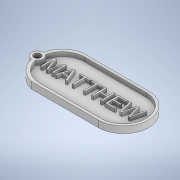
# Autodesk Inventor part: name_tag
Saved by Autodesk Inventor 2020 (Build 240168000, 168)
## iProperties
Created: 2022-11-14
Part Number: name_tag
Material: Generic
Document SubType Name: Modeling
Designer: Matthew Ng
Density: 1 g/cm^3
Appearance: Default
Author: Matthew Ng
Autodesk Inventor part; units mm, degrees
note: some values were not read from the file. Chosen so that the rebuilt part matches the saved one: direction of "Emboss1".
ref_plane "YZ Plane" through (0, 0, 0) normal (1, 0, 0) x (0, 1, 0)
ref_plane "XZ Plane" through (0, 0, 0) normal (0, 1, 0) x (-1, 0, 0)
ref_plane "XY Plane" through (0, 0, 0) normal (0, 0, 1) x (1, 0, 0)
sketch "Sketch1" plane through (0, 0, 0) normal (0, 1, 0) x (-1, 0, 0)
  line L0 (-15, 0) -> (-55, 0)
  line L1 (-55, -30) -> (-15, -30)
  arc A0 (-55, 0) -> (-55, -30) centre (-55, -15) ccw
  line L2 (-18.5, -1.5) -> (-55, -1.5)
  line L3 (-55, -28.5) -> (-18.5, -28.5)
  arc A1 (-55, -1.5) -> (-55, -28.5) centre (-55, -15) ccw
  circle A2 centre (-3.5, -15) radius 2
  circle A3 centre (-3.5, -15) radius 3.5
  arc A4 (-18.5, -28.5) -> (-5.3333, -17.9814) centre (-18.5, -15) ccw
  arc A5 (-5.3333, -12.0186) -> (-18.5, -1.5) centre (-18.5, -15) ccw
  arc A6 (-15, -30) -> (-3.5, -18.5) centre (-18.5, -15) ccw
  arc A7 (-3.5, -11.5) -> (-15, 0) centre (-18.5, -15) ccw
  point P0 (0, 0)
  point P1 (-35, -15)
  dimension "d2" = 30
  dimension "d8" = 7
  dimension "d9" = 4
  dimension "d28" = 27
  dimension "d29" = 70
  constraints: 16 point on circle, 8 centre point, 8 end point, 4 tangent, 2 parallel, 1 coincident, 1 horizontal
  measures "d2" distance between parallel lines of L0 L1
  measures "d8" diameter of A3
  measures "d9" diameter of A2
  measures "d28" distance between parallel lines of L2 L3
extrude "Extrusion1" add sketch "Sketch1" along normal blind 1.5 contours A3 A4 L3 A1 L2 A5
extrude "Extrusion2" add sketch "Sketch1" along normal blind 4 contours A7 A3 A5 L2 A1 L3 A4 A6 L1 A0 L0 | A3
sketch "Sketch2" plane through (0, 1.5, 0) normal (0, 1, 0) x (1, 0, 0)
  line L0 (8.3363, 19.2426) -> (40.4919, 19.2426) construction
  line L1 (40.4919, 19.2426) -> (40.4919, 12.4999) construction
  line L2 (40.4919, 12.4999) -> (8.3363, 12.4999) construction
  line L3 (8.3363, 12.4999) -> (8.3363, 19.2426) construction
  line L4 (9.1656, 11.2426) -> (9.1656, 19.2426)
  line L5 (9.1656, 19.2426) -> (10.7571, 19.2426)
  line L6 (10.7571, 19.2426) -> (12.6534, 13.5779)
  spline S0 degree 2 poles (12.6534, 13.5779) (12.9156, 12.7852) (13.0376, 12.395) knots 0 0 0 1 1 1
  spline S1 degree 2 poles (13.0376, 12.395) (13.1717, 12.8279) (13.4644, 13.6755) knots 0 0 0 1 1 1
  line L7 (13.4644, 13.6755) -> (15.3851, 19.2426)
  line L8 (15.3851, 19.2426) -> (16.8059, 19.2426)
  line L9 (16.8059, 19.2426) -> (16.8059, 11.2426)
  line L10 (16.8059, 11.2426) -> (15.7876, 11.2426)
  line L11 (15.7876, 11.2426) -> (15.7876, 17.9377)
  line L12 (15.7876, 17.9377) -> (13.4522, 11.2426)
  line L13 (13.4522, 11.2426) -> (12.501, 11.2426)
  line L14 (12.501, 11.2426) -> (10.1839, 18.0535)
  line L15 (10.1839, 18.0535) -> (10.1839, 11.2426)
  line L16 (10.1839, 11.2426) -> (9.1656, 11.2426)
  line L17 (17.6351, 11.2426) -> (20.7083, 19.2426)
  line L18 (20.7083, 19.2426) -> (21.8546, 19.2426)
  line L19 (21.8546, 19.2426) -> (25.1229, 11.2426)
  line L20 (25.1229, 11.2426) -> (23.9156, 11.2426)
  line L21 (23.9156, 11.2426) -> (22.9888, 13.6633)
  line L22 (22.9888, 13.6633) -> (19.6351, 13.6633)
  line L23 (19.6351, 13.6633) -> (18.7571, 11.2426)
  line L24 (18.7571, 11.2426) -> (17.6351, 11.2426)
  line L25 (19.94, 14.523) -> (22.6595, 14.523)
  line L26 (22.6595, 14.523) -> (21.8181, 16.7426)
  spline S2 degree 2 poles (21.8181, 16.7426) (21.44, 17.7548) (21.2571, 18.4011) knots 0 0 0 1 1 1
  spline S3 degree 2 poles (21.2571, 18.4011) (21.0985, 17.6328) (20.8242, 16.8706) knots 0 0 0 1 1 1
  line L27 (20.8242, 16.8706) -> (19.94, 14.523)
  line L28 (28.001, 11.2426) -> (28.001, 18.2974)
  line L29 (28.001, 18.2974) -> (25.3668, 18.2974)
  line L30 (25.3668, 18.2974) -> (25.3668, 19.2426)
  line L31 (25.3668, 19.2426) -> (31.7083, 19.2426)
  line L32 (31.7083, 19.2426) -> (31.7083, 18.2974)
  line L33 (31.7083, 18.2974) -> (29.062, 18.2974)
  line L34 (29.062, 18.2974) -> (29.062, 11.2426)
  line L35 (29.062, 11.2426) -> (28.001, 11.2426)
  line L36 (34.8303, 11.2426) -> (34.8303, 18.2974)
  line L37 (34.8303, 18.2974) -> (32.1961, 18.2974)
  line L38 (32.1961, 18.2974) -> (32.1961, 19.2426)
  line L39 (32.1961, 19.2426) -> (38.5376, 19.2426)
  line L40 (38.5376, 19.2426) -> (38.5376, 18.2974)
  line L41 (38.5376, 18.2974) -> (35.8912, 18.2974)
  line L42 (35.8912, 18.2974) -> (35.8912, 11.2426)
  line L43 (35.8912, 11.2426) -> (34.8303, 11.2426)
  line L44 (39.6656, 11.2426) -> (39.6656, 19.2426)
  line L45 (39.6656, 19.2426) -> (40.7266, 19.2426)
  line L46 (40.7266, 19.2426) -> (40.7266, 15.956)
  line L47 (40.7266, 15.956) -> (44.8729, 15.956)
  line L48 (44.8729, 15.956) -> (44.8729, 19.2426)
  line L49 (44.8729, 19.2426) -> (45.9339, 19.2426)
  line L50 (45.9339, 19.2426) -> (45.9339, 11.2426)
  line L51 (45.9339, 11.2426) -> (44.8729, 11.2426)
  line L52 (44.8729, 11.2426) -> (44.8729, 15.0108)
  line L53 (44.8729, 15.0108) -> (40.7266, 15.0108)
  line L54 (40.7266, 15.0108) -> (40.7266, 11.2426)
  line L55 (40.7266, 11.2426) -> (39.6656, 11.2426)
  line L56 (47.7205, 11.2426) -> (47.7205, 19.2426)
  line L57 (47.7205, 19.2426) -> (53.5132, 19.2426)
  line L58 (53.5132, 19.2426) -> (53.5132, 18.2974)
  line L59 (53.5132, 18.2974) -> (48.7815, 18.2974)
  line L60 (48.7815, 18.2974) -> (48.7815, 15.8523)
  line L61 (48.7815, 15.8523) -> (53.2144, 15.8523)
  line L62 (53.2144, 15.8523) -> (53.2144, 14.9072)
  line L63 (53.2144, 14.9072) -> (48.7815, 14.9072)
  line L64 (48.7815, 14.9072) -> (48.7815, 12.1877)
  line L65 (48.7815, 12.1877) -> (53.6961, 12.1877)
  line L66 (53.6961, 12.1877) -> (53.6961, 11.2426)
  line L67 (53.6961, 11.2426) -> (47.7205, 11.2426)
  line L68 (56.5498, 11.2426) -> (54.4278, 19.2426)
  line L69 (54.4278, 19.2426) -> (55.5132, 19.2426)
  line L70 (55.5132, 19.2426) -> (56.7327, 13.9987)
  spline S4 degree 2 poles (56.7327, 13.9987) (56.9278, 13.1755) (57.0742, 12.3584) knots 0 0 0 1 1 1
  spline S5 degree 2 poles (57.0742, 12.3584) (57.379, 13.645) (57.4339, 13.8401) knots 0 0 0 1 1 1
  line L71 (57.4339, 13.8401) -> (58.9522, 19.2426)
  line L72 (58.9522, 19.2426) -> (60.2327, 19.2426)
  line L73 (60.2327, 19.2426) -> (61.379, 15.1938)
  spline S6 degree 2 poles (61.379, 15.1938) (61.7998, 13.6877) (62.001, 12.3584) knots 0 0 0 1 1 1
  spline S7 degree 2 poles (62.001, 12.3584) (62.1534, 13.1206) (62.3973, 14.1023) knots 0 0 0 1 1 1
  line L74 (62.3973, 14.1023) -> (63.6473, 19.2426)
  line L75 (63.6473, 19.2426) -> (64.7144, 19.2426)
  line L76 (64.7144, 19.2426) -> (62.5315, 11.2426)
  line L77 (62.5315, 11.2426) -> (61.4949, 11.2426)
  line L78 (61.4949, 11.2426) -> (59.8242, 17.3401)
  spline S8 degree 2 poles (59.8242, 17.3401) (59.6046, 18.1023) (59.5681, 18.2791) knots 0 0 0 1 1 1
  spline S9 degree 2 poles (59.5681, 18.2791) (59.4339, 17.7304) (59.3303, 17.3401) knots 0 0 0 1 1 1
  line L79 (59.3303, 17.3401) -> (57.6412, 11.2426)
  line L80 (57.6412, 11.2426) -> (56.5498, 11.2426)
  point P0 (0, 0)
  constraints: 2 other
emboss "Emboss1" sketch "Sketch2" operation add depth 2 direction (0, -1, 0)
body "Solid1"
